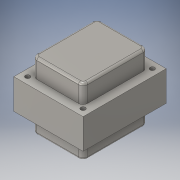
# Autodesk Inventor part: xmfr power
Saved by Autodesk Inventor 2016 (Build 200138000, 138)
## iProperties
Created: 2015-10-14
Part Number: xmfr power
Material: Iron, Malleable
Document SubType Name: Modeling
Designer: jeremyhale
Density: 7.15 g/cm^3
Appearance: Semi-Polished
Author: jeremyhale
Autodesk Inventor part; units mm, degrees
ref_plane "YZ Plane" through (0, 0, 0) normal (1, 0, 0) x (0, 1, 0)
ref_plane "XZ Plane" through (0, 0, 0) normal (0, 1, 0) x (-1, 0, 0)
ref_plane "XY Plane" through (0, 0, 0) normal (0, 0, 1) x (1, 0, 0)
sketch "Sketch1" plane through (0, 0, 0) normal (0, 1, 0) x (-1, 0, 0)
  line L0 (-47.625, 57.15) -> (47.625, 57.15)
  line L1 (47.625, 57.15) -> (47.625, -57.15)
  line L2 (47.625, -57.15) -> (-47.625, -57.15)
  line L3 (-47.625, -57.15) -> (-47.625, 57.15)
  line L4 (-47.625, 57.15) -> (47.625, -57.15) construction
  line L5 (47.625, 57.15) -> (-47.625, -57.15) construction
  point P0 (0, 0)
  dimension "d0" = 114.3
  dimension "d1" = 95.25
  constraints: 12 end point, 2 midpoint, 2 parallel, 1 horizontal, 1 perpendicular
  measures "d0" distance of L0.end L1.end
  measures "d1" distance of L1.end L2.end
extrude "Extrusion1" add sketch "Sketch1" along normal blind 41.275
sketch "Sketch2" plane through (0, 41.275, 0) normal (0, 1, 0) x (1, 0, 0)
  line L0 (28.575, -44.45) -> (-28.575, -44.45)
  line L1 (-34.925, -38.1) -> (-34.925, 38.1)
  line L2 (-28.575, 44.45) -> (28.575, 44.45)
  line L3 (34.925, 38.1) -> (34.925, -38.1)
  line L4 (34.925, -44.45) -> (-34.925, 44.45) construction
  line L5 (-34.925, -44.45) -> (34.925, 44.45) construction
  arc A0 (-34.925, -38.1) -> (-28.575, -44.45) centre (-28.575, -38.1) ccw
  arc A1 (-28.575, 44.45) -> (-34.925, 38.1) centre (-28.575, 38.1) ccw
  arc A2 (34.925, 38.1) -> (28.575, 44.45) centre (28.575, 38.1) ccw
  arc A3 (28.575, -44.45) -> (34.925, -38.1) centre (28.575, -38.1) ccw
  line L6 (-47.625, 57.15) -> (-47.625, -57.15) projected
  line L7 (47.625, 57.15) -> (-47.625, 57.15) projected
  point P0 (0, 0)
  dimension "d6" = 6.35
  dimension "d25" = 12.7
  dimension "d26" = 12.7
  constraints: 12 end point, 8 point on circle, 8 point on line, 8 tangent, 4 centre point, 3 equal radius, 2 midpoint, 2 parallel, 1 horizontal, 1 perpendicular
  measures "d6" radius of A0
  measures "d25" distance between parallel lines of L6 L1
  measures "d26" distance between parallel lines of L2 L7
extrude "Extrusion2" add sketch "Sketch2" along normal blind 25.4
fillet "Fillet1" radius 3.175 8 edges at (33.0651, 66.675, 42.5901) (34.925, 66.675, 0) (33.0651, 66.675, -42.5901) (0, 66.675, -44.45) (-33.0651, 66.675, -42.5901) (-34.925, 66.675, 0) (-33.0651, 66.675, 42.5901) (0, 66.675, 44.45)
hole "Hole1" at (38.1, 41.275, 47.625) direction (0, -1, 0) diameter 6.35 end through all
pattern_linear "Rectangular Pattern1" count 2 spacing 95.25 along (0, 0, -1) count 2 spacing 76.2 along (-1, 0, 0) of "Hole1"
sketch "Sketch3" plane through (0, 0, 0) normal (0, -1, 0) x (1, 0, 0)
  line L0 (-28.575, -44.45) -> (28.575, -44.45)
  line L1 (34.925, -38.1) -> (34.925, 38.1)
  line L2 (28.575, 44.45) -> (-28.575, 44.45)
  line L3 (-34.925, 38.1) -> (-34.925, -38.1)
  line L4 (-34.925, -44.45) -> (34.925, 44.45) construction
  line L5 (34.925, -44.45) -> (-34.925, 44.45) construction
  line L6 (47.625, 57.15) -> (-47.625, 57.15) projected
  line L7 (47.625, -57.15) -> (47.625, 57.15) projected
  arc A0 (-28.575, 44.45) -> (-34.925, 38.1) centre (-28.575, 38.1) ccw
  arc A1 (34.925, 38.1) -> (28.575, 44.45) centre (28.575, 38.1) ccw
  arc A2 (28.575, -44.45) -> (34.925, -38.1) centre (28.575, -38.1) ccw
  arc A3 (-34.925, -38.1) -> (-28.575, -44.45) centre (-28.575, -38.1) ccw
  point P0 (0, 0)
  dimension "d27" = 12.7
  dimension "d28" = 12.7
  dimension "d29" = 6.35
  constraints: 12 end point, 8 point on circle, 8 point on line, 8 tangent, 4 centre point, 3 equal radius, 2 midpoint, 2 parallel, 1 horizontal, 1 perpendicular
  measures "d27" distance between parallel lines of L2 L6
  measures "d28" distance between parallel lines of L7 L1
  measures "d29" radius of A0
extrude "Extrusion3" add sketch "Sketch3" along normal blind 25.4
fillet "Fillet2" radius 3.175 8 edges at (-33.0651, -25.4, 42.5901) (-34.925, -25.4, 0) (-33.0651, -25.4, -42.5901) (0, -25.4, -44.45) (33.0651, -25.4, -42.5901) (34.925, -25.4, 0) (33.0651, -25.4, 42.5901) (0, -25.4, 44.45)
body "Solid1"
